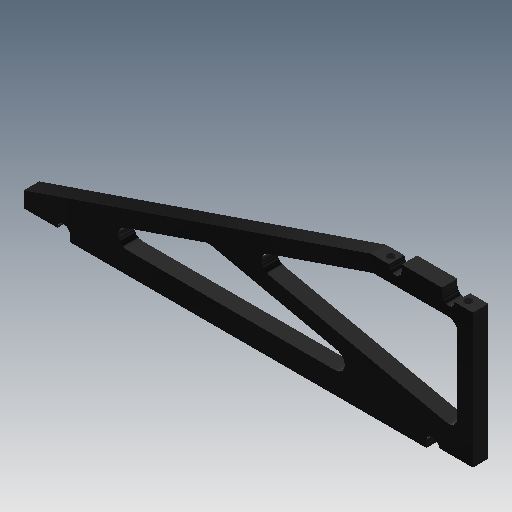
# Autodesk Inventor part: 前腕_サブフレーム_1_1
Saved by Autodesk Inventor 2017.3 (Build 213256000, 256)
## iProperties
Created: 2016-05-04
Part Number: 前腕_サブフレーム_1_1
Material: アセタール樹脂、黒
Document SubType Name: Modeling
Designer: hiroaki
Density: 1.425 g/cm^3
Appearance: 滑らか - 黒
Mass: 16.6655 g
Surface Area: 81.5563 cm^2
Volume: 11.6951 cm^3
Author: hiroaki
Autodesk Inventor part; units mm, degrees
ref_plane "YZ Plane" through (0, 0, 0) normal (1, 0, 0) x (0, 1, 0)
ref_plane "XZ Plane" through (0, 0, 0) normal (0, 1, 0) x (-1, 0, 0)
ref_plane "XY Plane" through (0, 0, 0) normal (0, 0, 1) x (1, 0, 0)
sketch "スケッチ1" plane through (0, 0, 0) normal (0, 0, 1) x (1, 0, 0)
  line L0 (-72.5, -21.65) -> (72.5, -21.65) construction
  line L1 (72.5, -21.65) -> (72.5, 21.65) construction
  line L2 (72.5, 21.65) -> (-72.5, 21.65) construction
  line L3 (-72.5, 21.65) -> (-72.5, -21.65) construction
  line L4 (-72.5, -21.65) -> (72.5, 21.65) construction
  line L5 (72.5, -21.65) -> (-72.5, 21.65) construction
  line L6 (-67.5, 21.65) -> (-67.5, -21.65) construction
  line L7 (0, 0) -> (0, 21.65) construction
  line L8 (0, 0) -> (-72.5, 0) construction
  line L9 (67.5, 21.65) -> (67.5, -21.65) construction
  line L10 (-72.5, -21.65) -> (-61.6, -21.65)
  line L11 (49.5, 21.65) -> (49.5, 23.65)
  line L12 (49.5, 23.65) -> (62.5, 23.65)
  line L13 (62.5, 23.65) -> (62.5, 21.65)
  line L14 (66.6, 21.65) -> (72.5, 21.65)
  line L15 (72.5, 21.65) -> (72.5, -21.65)
  line L16 (72.5, -21.65) -> (61.6, -21.65)
  line L17 (-57.5, -21.65) -> (-57.5, -23.65)
  line L18 (-57.5, -23.65) -> (57.5, -23.65)
  line L19 (57.5, -23.65) -> (57.5, -21.65)
  arc A0 (45.4, 21.65) -> (49.5, 21.65) centre (47.45, 21.65) ccw
  arc A1 (62.5, 21.65) -> (66.6, 21.65) centre (64.55, 21.65) ccw
  arc A2 (-57.5, -21.65) -> (-61.6, -21.65) centre (-59.55, -21.65) ccw
  arc A3 (61.6, -21.65) -> (57.5, -21.65) centre (59.55, -21.65) ccw
  line L20 (-72.5, -21.65) -> (-72.5, -16.65)
  line L21 (-72.5, -16.65) -> (39.5, 21.65)
  line L22 (45.4, 21.65) -> (39.5, 21.65)
  line L23 (66.95, 24.476) -> (70.05, 24.476) construction
  line L24 (70.05, 24.476) -> (70.05, 13.3235) construction
  line L25 (70.05, 13.3235) -> (66.95, 13.3235) construction
  line L26 (66.95, 13.3235) -> (66.95, 24.476) construction
  line L27 (68.5, 24.476) -> (68.5, 13.3235) construction
  line L28 (41.95, 24.476) -> (45.05, 24.476) construction
  line L29 (45.05, 24.476) -> (45.05, 13.9945) construction
  line L30 (45.05, 13.9945) -> (41.95, 13.9945) construction
  line L31 (41.95, 13.9945) -> (41.95, 24.476) construction
  line L32 (43.5, 24.476) -> (43.5, 13.9945) construction
  dimension "d16" = 5
  dimension "d20" = 43.3
  dimension "d40" = 135
  dimension "d41" = 10
  dimension "d42" = 2.05
  dimension "d43" = 2
  dimension "d44" = 5
  dimension "d45" = 10
  dimension "d46" = 10
  dimension "d48" = 3.1
  dimension "d50" = 4
  dimension "d51" = 25
  dimension "d52" = 3.1
  dimension "d62" = 6
  dimension "d63" = 6
  constraints: 66 end point, 11 perpendicular, 8 midpoint, 8 point on circle, 6 parallel, 6 point on line, 5 collinear, 4 centre point, 4 horizontal, 4 horizontal alignment, 3 equal radius, 3 tangent, 2 symmetric about line, 2 vertical, 3 other
  measures "d16" distance between parallel lines of L3 L6
  measures "d20" distance of L2.end L0.start
  measures "d40" distance between parallel lines of L9 L6
  measures "d41" distance between parallel lines of L6 L17
  measures "d42" radius of A2
  measures "d43" distance between parallel lines of L0 L18
  measures "d44" distance from line of L10 L20.end
  measures "d45" distance between parallel lines of L1 L13
  measures "d46" distance from line of L21.end L11
  measures "d48" distance of L23.start L23.end
  measures "d50" distance between parallel lines of L1 L27
  measures "d51" distance between parallel lines of L27 L32
  measures "d52" distance of L28.start L28.end
  measures "d62" distance between parallel lines of L13 L27
  measures "d63" distance between parallel lines of L32 L11
extrude "押し出し1" add sketch "スケッチ1" along normal blind 2.5
mirror "ミラー1" about plane through (8.3734, -6.8299, 0) normal (0, 0, -1) of "押し出し1"
sketch "スケッチ2" plane through (-72.5, -21.65, 2.5) normal (0, -1, 0) x (1, 0, 0)
  line L0 (0, -5) -> (0, 0)
  line L1 (15, -5) -> (130, -5) construction
  line L2 (72.5, -5) -> (72.5, 0) construction
  line L3 (15, 0) -> (130, 0) construction
  point P0 (72.5, -2.5)
  point P1 (5, -2.5)
  point P2 (140, -2.5)
  point P3 (0, -2.5)
  dimension "d26" = 5
  constraints: 4 end point, 3 midpoint, 2 horizontal alignment, 1 symmetric about line
  measures "d26" distance from line of point (5, -2.5) L0
hole "穴1" at (-67.5, -21.65, 0) at (67.5, -21.65, 0) direction (0, 1, 0) diameter 2.459 depth 2 thread size "M3x0.5" class "6H" standard "ISO Metric profile"
sketch "スケッチ4" plane through (66.6, 21.65, 2.5) normal (0, 1, 0) x (1, 0, 0)
  line L0 (5.9, 5) -> (5.9, 0) projected
  point P0 (-66.6, 2.5)
  point P1 (1.9, 2.5)
  point P2 (-23.1, 2.5)
  point P3 (5.9, 2.5)
  dimension "d53" = 4
  dimension "d54" = 25
  constraints: 2 horizontal alignment, 1 midpoint
  measures "d53" distance from line of point (1.9, 2.5) L0
  measures "d54" distance of point (-23.1, 2.5) point (1.9, 2.5)
hole "穴2" at (68.5, 21.65, 0) at (43.5, 21.65, 0) direction (0, -1, 0) diameter 2.459 depth 2.5 thread size "M3x0.5" class "6H" standard "ISO Metric profile"
sketch "スケッチ6" plane through (0, 0, 2.5) normal (0, 0, 1) x (1, 0, 0)
  line L0 (61.6, -21.65) -> (72.5, -21.65) projected
  line L1 (72.5, -21.65) -> (72.5, 21.65) projected
  line L2 (72.5, 21.65) -> (66.6, 21.65) projected
  line L3 (39.5, 21.65) -> (-72.5, -16.65) projected
  line L4 (67.5, 16.65) -> (67.5, -16.65) construction
  line L5 (67.5, -16.65) -> (-57.0473, -16.65) construction
  line L6 (-57.0473, -16.65) -> (40.3313, 16.65) construction
  line L7 (40.3313, 16.65) -> (67.5, 16.65) construction
  line L8 (67.5, -16.65) -> (-8.358, 0) construction
  line L9 (67.5, -14.0905) -> (67.5, 16.65)
  line L10 (67.5, 16.65) -> (40.3313, 16.65)
  line L11 (40.3313, 16.65) -> (-3.7993, 1.5589)
  line L12 (-3.7993, 1.5589) -> (67.5, -14.0905)
  line L13 (55.8388, -16.65) -> (-57.0473, -16.65)
  line L14 (-57.0473, -16.65) -> (-12.9167, -1.5589)
  line L15 (-12.9167, -1.5589) -> (55.8388, -16.65)
  point P0 (0, 0)
  dimension "d72" = 5
  dimension "d73" = 5
  dimension "d74" = 5
  dimension "d75" = 5
  dimension "d76" = 5
  constraints: 24 end point, 5 collinear, 3 parallel, 2 horizontal, 2 perpendicular, 2 vertical, 1 midpoint, 1 other
  measures "d72" distance between parallel lines of L7 L2
  measures "d73" distance between parallel lines of L0 L5
  measures "d74" distance between parallel lines of L1 L4
  measures "d75" distance between parallel lines of L3 L6
  measures "d76" distance between parallel lines of L15 L12
extrude "押し出し4" cut sketch "スケッチ6" against normal blind 10
fillet "フィレット3" radius 3 7 edges at (-3.7993, 1.5589, 0) (40.3313, 16.65, 0) (67.5, -14.0905, 0) (55.8388, -16.65, 0) (-12.9167, -1.5589, 0) (-57.0473, -16.65, 0) (67.5, 16.65, 0)
equation "\"d16\" = d4"
equation "\"d40\" = d6"
equation "\"d41\" = d3"
equation "\"d46\" = d45"
equation "\"d63\" = d62"
equation "\"d26\" = d4"
equation "\"d53\" = d50"
equation "\"d54\" = d51"
equation "\"d73\" = d72"
equation "\"d74\" = d73"
equation "\"d75\" = d74"
equation "\"d76\" = d74"
equation "\"d4\" = 5"
equation "\"d6\" = 135"
equation "\"d3\" = 10"
